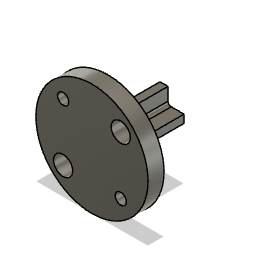
cross_peg (Autodesk Fusion 360 design; units mm, degrees)
Autodesk Fusion 360 part; units mm, degrees
sketch "Sketch1" plane through (0, 0, 0) normal (0, 0, 1) x (1, 0, 0)
  circle A0 centre (0, 0) radius 35
  circle A1 centre (18, 18) radius 3.5
  circle A2 centre (-18, -18) radius 3.5
  circle A3 centre (-18, 18) radius 6
  circle A4 centre (18, -18) radius 6
  dimension "d1" = 70
  dimension "d2" = 7
  dimension "d3" = 18
  dimension "d4" = 18
  dimension "d5" = 7
  dimension "d6" = 18
  dimension "d7" = 18
  dimension "d8" = 12
  dimension "d9" = 18
  dimension "d10" = 18
  dimension "d11" = 12
  dimension "d12" = 18
  dimension "d13" = 18
  constraint coincident A0.centre origin
  measures "d1" diameter of A0
  measures "d2" diameter of A1
  measures "d3" horizontal distance of A0.centre A1.centre
  measures "d4" vertical distance of A0.centre A1.centre
  measures "d5" diameter of A2
  measures "d6" vertical distance of A0.centre A2.centre
  measures "d7" horizontal distance of A0.centre A2.centre
  measures "d8" diameter of A3
  measures "d9" horizontal distance of A0.centre A3.centre
  measures "d10" vertical distance of A0.centre A3.centre
  measures "d11" diameter of A4
  measures "d12" vertical distance of A0.centre A4.centre
  measures "d13" horizontal distance of A0.centre A4.centre
extrude "Extrude1" add sketch "Sketch1" against normal blind 10 makes body 1
sketch "Sketch2" plane through (0, 0, 0) normal (0, 0, 1) x (1, 0, 0)
  line L0 (12.5, 12.5) -> (-12.5, 12.5)
  line L1 (-12.5, 12.5) -> (-12.5, -12.5)
  line L2 (-12.5, -12.5) -> (12.5, -12.5)
  line L3 (12.5, -12.5) -> (12.5, 12.5)
  line L4 (12.5, 12.5) -> (-12.5, -12.5) construction
  line L5 (-12.5, 12.5) -> (12.5, -12.5) construction
  dimension "d16" = 25
  dimension "d17" = 25
  constraint horizontal L0
  constraint perpendicular L0 L1
  constraint parallel L0 L2
  constraint parallel L1 L3
  constraint coincident L4 origin
  constraint coincident L5 origin
  measures "d16" distance of L0.end L1.end
  measures "d17" distance of L1.end L2.end
extrude "Extrude2" add sketch "Sketch2" along normal blind 10 bodies 1
sketch "Sketch3" plane through (0, 0, 10) normal (0, 0, 1) x (1, 0, 0)
  line L0 (12.5, -12.5) -> (12.5, 12.5)
  line L1 (12.5, 12.5) -> (-12.5, 12.5)
  line L2 (-12.5, 12.5) -> (-12.5, -12.5)
  line L3 (-12.5, -12.5) -> (12.5, -12.5)
  line L4 (2.5, 12.5) -> (-2.5, 12.5)
  line L5 (-2.5, 12.5) -> (-2.5, -12.5)
  line L6 (-2.5, -12.5) -> (2.5, -12.5)
  line L7 (2.5, -12.5) -> (2.5, 12.5)
  line L8 (2.5, 12.5) -> (-2.5, -12.5) construction
  line L9 (-2.5, 12.5) -> (2.5, -12.5) construction
  line L10 (12.5, -2.5) -> (-12.5, -2.5)
  line L11 (-12.5, -2.5) -> (-12.5, 2.5)
  line L12 (-12.5, 2.5) -> (12.5, 2.5)
  line L13 (12.5, 2.5) -> (12.5, -2.5)
  line L14 (12.5, -2.5) -> (-12.5, 2.5) construction
  line L15 (-12.5, -2.5) -> (12.5, 2.5) construction
  dimension "d20" = 5
  dimension "d21" = 5
  constraint horizontal L4
  constraint perpendicular L4 L5
  constraint parallel L4 L6
  constraint parallel L5 L7
  constraint coincident L8 origin
  constraint coincident L9 origin
  constraint coincident L1 L4.start
  constraint horizontal L10
  constraint perpendicular L10 L11
  constraint parallel L10 L12
  constraint parallel L11 L13
  constraint coincident L14 origin
  constraint coincident L15 origin
  constraint coincident L0 L10.start
  measures "d20" distance of L10 L12
  measures "d21" distance of L5 L7
extrude "Extrude3" add sketch "Sketch3" along normal blind 25 contours L0 L7 L10 L12 L13 | L3 L5 L6 L7 L10 | L5 L7 L10 L12 | L1 L4 L5 L7 L12 | L2 L5 L10 L11 L12 bodies 1
fillet "Fillet1" radius 2 4 edges at (2.5, -2.5, 22.5) (2.5, 2.5, 22.5) (-2.5, 2.5, 22.5) (-2.5, -2.5, 22.5) on bodies 1
split "Split1" by plane through (0, 0, 0) normal (0, 0, 1) bodies 1 makes body 2 at (12.5, 0.8333, 3.3333)
split "Split2" by plane through (0, 0, 10) normal (0, 0, 1) bodies 2 makes body 3 at (0.9962, -0.9289, 35)
split "Split3" by plane through (2.5, 2.5, 10) normal (1, 0, 0) bodies 3 makes body 4 at (9.8333, -2.5, 18.3333)
split "Split4" by plane through (-2.5, 12.5, 10) normal (-1, 0, 0) bodies 3 makes body 5 at (-7.1667, -2.5, 18.3333)
split "Split5" by plane through (2.5, 2.5, 10) normal (0, 1, 0) bodies 4 makes body 6 at (3.5835, 2.7223, 18.3333)
split "Split6" by plane through (12.5, -2.5, 10) normal (0, -1, 0) bodies 4 makes body 7 at (2.5023, -4.4048, 18.3333)
split "Split7" by plane through (-2.5, -2.5, 10) normal (0, -1, 0) bodies 5 makes body 8 at (-2.5023, -4.4048, 18.3333)
split "Split8" by plane through (-12.5, 2.5, 10) normal (0, 1, 0) bodies 5 makes body 9 at (-4.4048, 2.5023, 18.3333)
move_body "Move1" bodies 7 3 8 5 4 6 2 9 1 to x (1, 0, 0) y (0, -1, 0) z (0, 0, -1) at (0, 0, 0)
move_body "Move2" bodies 7 9 2 8 5 4 3 1 6 to x (1, 0, 0) y (0, 1, 0) z (0, 0, 1) at (0, 0, 10)
